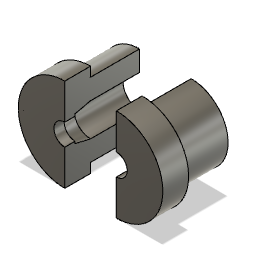
sensor_housing (Autodesk Fusion 360 design; units mm, degrees)
Autodesk Fusion 360 part; units mm, degrees
sketch "Sketch1" plane through (0, 0, 0) normal (0, 0, 1) x (1, 0, 0)
  arc A0 (-100, 7.15) -> (-100, -7.15) centre (-100, 0) ccw
  line L0 (-100, 7.15) -> (-100, -7.15)
  arc A1 (-100, 3.2) -> (-100, -3.2) centre (-100, 0) ccw
  dimension "d17" = 3.2
  dimension "d18" = 7.15
  constraint vertical L0
  constraint coincident L0 A1.end
  constraint coincident L0 A1.start
  constraint coincident A0.centre A1.centre
  measures "d17" radius of A1
  measures "d18" radius of A0
extrude "Extrude1" add sketch "Sketch1" along normal blind 9.5 contours A0 L0 A1 makes body 1
sketch "Sketch2" plane through (0, 0, 9.5) normal (0, 0, 1) x (1, 0, 0)
  line L0 (-100, -7.15) -> (-100, -3.2)
  line L1 (-100, 3.2) -> (-100, 7.15)
  arc A0 (-100, 2.5) -> (-100, -2.5) centre (-100, 0) ccw
  line L2 (-100, 2.5) -> (-100, -2.5)
  arc A1 (-100, 9) -> (-100, -9) centre (-100, 0) ccw
  line L3 (-100, -9) -> (-100, 9)
  dimension "d19" = 2.5
  dimension "d22" = 9
  constraint coincident A0.centre A1.centre
  constraint vertical L3
  measures "d19" radius of A0
  measures "d22" radius of A1
extrude "Extrude2" add sketch "Sketch2" along normal blind 3 contours L0 L1 A0 A1 L3 bodies 1
sketch "Sketch3" plane through (0, 0, 12.5) normal (0, 0, 1) x (1, 0, 0)
  line L0 (-100, -9) -> (-100, -2.5)
  line L1 (-100, 2.5) -> (-100, 9)
  arc A0 (-100, 9) -> (-100, -9) centre (-100, 0) ccw
  line L2 (-100, -9) -> (-100, 9)
  arc A1 (-100, 2.1) -> (-100, -2.1) centre (-100, 0) ccw
  line L3 (-100, -2.1) -> (-100, 2.1)
  arc A2 (-100, 9) -> (-100, -9) centre (-100, 0) ccw
  arc A3 (-100, 9) -> (-100, -9) centre (-100, 0) ccw
  dimension "d20" = 2.1
  dimension "d21" = 85
  constraint coincident L0.start A0.end
  constraint coincident L1.end A0.start
  constraint coincident L2 A1.end
  constraint coincident L2 A1.start
  measures "d20" radius of A1
extrude "Extrude3" add sketch "Sketch3" along normal blind 2 contours L0 L1 A0 L2 A1 A2 A3 bodies 1
mirror "Mirror1" about plane through (0, 0, 0) normal (1, 0, 0) of bodies 1 makes body 2
sketch "Sketch4" plane through (-100, 0, 0) normal (1, 0, 0) x (0, 0, -1)
  line L0 (-9.5, 3.2) -> (0, 3.2)
  line L1 (0, 3.2) -> (0, 7.15)
  line L2 (0, 7.15) -> (-9.5, 7.15)
  line L3 (-9.5, 7.15) -> (-9.5, 9)
  line L4 (-9.5, 9) -> (-14.5, 9)
  line L5 (-14.5, 9) -> (-14.5, 2.1)
  line L6 (-14.5, 9) -> (-14.5, -9) construction
  line L7 (0, 0) -> (-14.5, 0) construction
  line L8 (-12.5, 2.5) -> (-9.5, 2.5)
  line L9 (-9.5, 2.5) -> (-9.5, 3.2)
  line L10 (-14.5, 2.1) -> (-12.5, 2.1)
  line L11 (-12.5, 2.1) -> (-12.5, 2.5)
  constraint coincident L7.start origin
  constraint midpoint L6 L7.end
hole "Hole1" at (-109, 0, 13.8909) direction (1, 0, 0) diameter 1 depth 1 tip angle 118 bodies 1
loft "Loft3" cut section 1 face at (-100.1595, 3.196, 3.1667) section 2 face at (-101.3036, 2.1332, 11.5) on bodies 1 bodies 1
move_body "Move1" bodies 1 to x (1, 0, 0) y (0, 1, 0) z (0, 0, 1) at (190, 0, 0)
equation "d18 = ( 14.5 / 2 ) * 1 mm - 0.1 mm"
